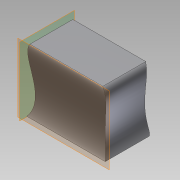
# Autodesk Inventor part: 0603 board
Saved by Autodesk Inventor 2011 (Build 150239000, 239)
## iProperties
Created: 2010-12-28
Part Number: 0603 board
Document SubType Name: Modeling
Designer: abbath
Density: 1 g/cm^3
Author: abbath
Autodesk Inventor part; units mm, degrees
ref_plane "YZ Plane" through (0, 0, 0) normal (1, 0, 0) x (0, 1, 0)
ref_plane "XZ Plane" through (0, 0, 0) normal (0, 1, 0) x (-1, 0, 0)
ref_plane "XY Plane" through (0, 0, 0) normal (0, 0, 1) x (1, 0, 0)
sketch "Эскиз1" plane through (0, 0, 0) normal (0, 0, 1) x (1, 0, 0)
  line L0 (-1, -0.6) -> (1, -0.6)
  line L1 (1, -0.6) -> (1, 0.6)
  line L2 (1, 0.6) -> (-1, 0.6)
  line L3 (-1, 0.6) -> (-1, -0.6)
  line L4 (-0.25, -0.4) -> (-0.25, 0.4) projected
  line L5 (-0.25, 0.4) -> (-0.8, 0.4) projected
  line L6 (-0.8, 0.4) -> (-0.8, -0.4) projected
  line L7 (-0.8, -0.4) -> (-0.25, -0.4) projected
  line L8 (0.25, 0.4) -> (0.25, -0.4) projected
  line L9 (0.25, -0.4) -> (0.8, -0.4) projected
  line L10 (0.8, -0.4) -> (0.8, 0.4) projected
  line L11 (0.8, 0.4) -> (0.25, 0.4) projected
  point P0 (0, 0)
  dimension "d0" = 0.2
  dimension "d1" = 0.2
  dimension "d2" = 0.2
  dimension "d3" = 0.2
  constraints: 8 end point, 2 parallel, 1 horizontal, 1 perpendicular
  measures "d0" distance between parallel lines of L3 L6
  measures "d1" distance between parallel lines of L2 L5
  measures "d2" distance between parallel lines of L1 L10
  measures "d3" distance between parallel lines of L0 L9
extrude "Выдавливание1" add sketch "Эскиз1" along normal blind 1.5 contours L3 L2 L1 L0 | L7 L6 L5 L4 | L11 L10 L9 L8
ref_plane "РабПлоскость1" through (-1, -0.6, 0) normal (0, -1, 0) x (1, 0, 0)
ref_plane "РабПлоскость2" through (-1, 0.6, 0) normal (-1, 0, 0) x (0, -1, 0)
sketch "Эскиз2" plane through (-1, -0.6, 0) normal (0, -1, 0) x (1, 0, 0)
  line L0 (2, 1.5) -> (0, 1.5) projected
  line L1 (0, 0) -> (0, 1.5) projected
  line L2 (0, 0) -> (2, 0) projected
  line L3 (2, 0) -> (2, 1.5) projected
  spline S0 degree 3 poles (1.9537, 0) (1.6088, 0.4735) (2.1515, 1.3588) (1.8533, 1.5) knots 0 0 0 0 1 1 1 1
  spline S1 degree 3 poles (0.0633, 0) (0.2846, 0.3099) (-0.0024, 1.179) (0.0963, 1.5) knots 0 0 0 0 1 1 1 1
  point P0 (1, 0)
  point P1 (1.8557, 0.6949)
  point P2 (1.9464, 1.311)
  point P3 (0.1493, 0.4099)
  point P4 (0.0882, 1.0857)
  constraints: 4 point on line, 8 other
extrude "Выдавливание2" cut sketch "Эскиз2" against normal through all contours L3 L2 S0 L0 | S1 L2 L1 L0
sketch "Эскиз3" plane through (-1, 0.6, 0) normal (-1, 0, 0) x (0, -1, 0)
  line L0 (0, 0) -> (0, 1.5) projected
  line L1 (1.2, 0) -> (0, 0) projected
  line L2 (1.2, 1.5) -> (1.2, 0) projected
  line L3 (0, 1.5) -> (1.2, 1.5) projected
  spline S0 degree 3 poles (1.1496, 0) (0.838, 0.3452) (1.2562, 1.3831) (1.1082, 1.5) knots 0 0 0 0 1 1 1 1
  spline S1 degree 3 poles (0.0904, 0) (-0.0812, 0.0387) (0.3049, 1.3936) (0.0735, 1.5) knots 0 0 0 0 1 1 1 1
  point P0 (0.6, 0)
  point P1 (1.0399, 0.6111)
  point P2 (1.1392, 1.3283)
  point P3 (0.0452, 0.1765)
  point P4 (0.1462, 1.1268)
  constraints: 4 point on line, 8 other
extrude "Выдавливание3" cut sketch "Эскиз3" against normal through all contours L0 L3 S1 L1 | S0 L3 L2 L1
